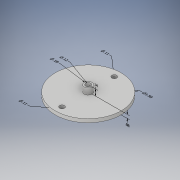
# Autodesk Inventor part: Servo Horn v1
Saved by Autodesk Inventor 2018 (Build 220112000, 112)
## iProperties
Created: 2019-12-10
Part Number: Servo Horn v1
Material: Generic
Document SubType Name: Modeling
Designer: AOFUser
Density: 1 g/cm^3
Appearance: Default
Author: AOFUser
Autodesk Inventor part; units mm, degrees
ref_plane "YZ Plane" through (0, 0, 0) normal (1, 0, 0) x (0, 1, 0)
ref_plane "XZ Plane" through (0, 0, 0) normal (0, 1, 0) x (-1, 0, 0)
ref_plane "XY Plane" through (0, 0, 0) normal (0, 0, 1) x (1, 0, 0)
sketch "Sketch1" plane through (0, 0, 0) normal (0, 1, 0) x (-1, 0, 0)
  circle A0 centre (0, 0) radius 19.05
  dimension "d0" = 38.1
  constraints: 1 centre point, 1 coincident
  measures "d0" diameter of A0
extrude "Extrusion1" add sketch "Sketch1" along normal blind 2.032
sketch "Sketch5" plane through (0, 2.032, 0) normal (0, 1, 0) x (1, 0, 0)
  circle A0 centre (0, 0) radius 2.286
  dimension "d14" = 4.572
  constraints: 1 centre point, 1 coincident
  measures "d14" diameter of A0
extrude "Extrusion3" add sketch "Sketch5" along normal blind 3.556
sketch "Sketch6" plane through (0, 5.588, 0) normal (0, 1, 0) x (1, 0, 0)
  circle A0 centre (0, 0) radius 1.4605
  dimension "d17" = 2.921
  constraints: 1 centre point, 1 coincident
  measures "d17" diameter of A0
extrude "Extrusion4" cut sketch "Sketch6" against normal blind 4.572
sketch "Sketch7" plane through (0, 1.016, 0) normal (0, 1, 0) x (1, 0, 0)
  circle A0 centre (0, 0) radius 1.016
  dimension "d20" = 2.032
  constraints: 1 centre point, 1 coincident
  measures "d20" diameter of A0
extrude "Extrusion5" cut sketch "Sketch7" against normal blind 4.572
sketch "Sketch8" plane through (0, 2.032, 0) normal (0, 1, 0) x (1, 0, 0)
  circle A0 centre (0, 0) radius 19.05 projected
  line L0 (0, 19.05) -> (0, 15.113)
  line L1 (0, -19.05) -> (0, -15.113)
  dimension "d23" = 3.937
  dimension "d24" = 3.937
  constraints: 4 end point, 2 point on circle, 2 vertical
  measures "d23" distance of L0.start L0.end
  measures "d24" distance of L1.start L1.end
hole "Hole2" at (0, 2.032, -15.113) direction (0, -1, 0) diameter 2.794 end through all
sketch "Sketch9" plane through (0, 2.032, 0) normal (0, 1, 0) x (1, 0, 0)
  circle A0 centre (0, 0) radius 19.05 projected
  line L0 (0, -19.05) -> (0, -15.113)
  dimension "d32" = 3.937
  constraints: 2 end point, 1 vertical, 1 vertical alignment, 1 other
  measures "d32" distance of L0.start L0.end
hole "Hole3" at (0, 2.032, 15.113) direction (0, -1, 0) diameter 2.794 end through all
body "Solid1"
